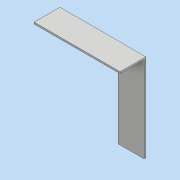
# Autodesk Inventor part: Giá đỡ 1
Saved by Autodesk Inventor 2018 (Build 220112000, 112)
## iProperties
Created: 2020-10-11
Part Number: Giá đỡ 1
Material: Generic
Document SubType Name: Modeling
Designer: ASUS
Density: 1 g/cm^3
Appearance: Default
Author: ASUS
Autodesk Inventor part; units mm, degrees
ref_plane "YZ Plane" through (0, 0, 0) normal (1, 0, 0) x (0, 1, 0)
ref_plane "XZ Plane" through (0, 0, 0) normal (0, 1, 0) x (-1, 0, 0)
ref_plane "XY Plane" through (0, 0, 0) normal (0, 0, 1) x (1, 0, 0)
sketch "Sketch1" plane through (0, 0, 0) normal (0, 1, 0) x (-1, 0, 0)
  line L0 (0, 0) -> (18, 0)
  line L1 (18, 0) -> (18, -60)
  line L2 (18, -60) -> (0, -60)
  line L3 (0, -60) -> (0, 0)
  dimension "d0" = 18
  dimension "d1" = 60
  constraints: 8 end point, 2 parallel, 1 horizontal, 1 perpendicular
  measures "d0" distance of L1.end L2.end
  measures "d1" distance of L0.end L1.end
extrude "Extrusion1" add sketch "Sketch1" along normal blind 1.2
sketch "Sketch3" plane through (-18, 0, 0) normal (0, 0, 1) x (1, 0, 0)
  line L0 (0, 1.2) -> (18, 1.2) projected
  line L1 (18, 1.2) -> (-42, 1.2)
  line L2 (-42, 1.2) -> (-42, -16.8)
  line L3 (-42, -16.8) -> (18, -16.8)
  line L4 (18, -16.8) -> (18, 1.2)
  point P0 (18, 0)
  dimension "d4" = 60
  dimension "d5" = 18
  constraints: 8 end point, 2 parallel, 1 horizontal, 1 perpendicular
  measures "d4" distance of L3.end L2.end
  measures "d5" distance of L2.end L1.end
extrude "Extrusion2" add sketch "Sketch3" along normal blind 1.2
body "Solid1"
